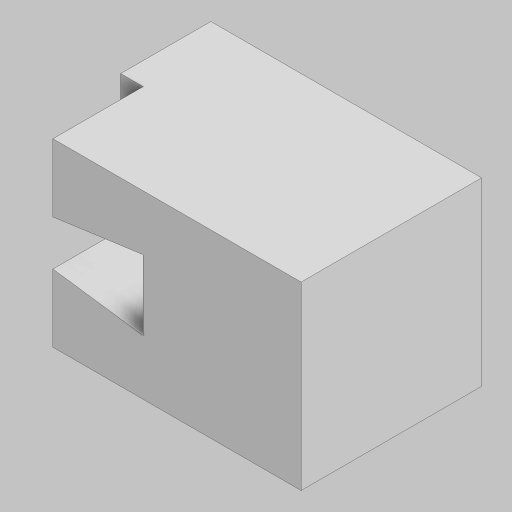
# Autodesk Inventor part: Hembra_parametrizada
Saved by Autodesk Inventor 2023 (Build 270158000, 158)
## iProperties
Created: 2026-02-22
Part Number: Hembra_parametrizada
Material: Genérico
Document SubType Name: Modeling
Designer: MARTIN MAESTRE
Density: 1 g/cm^3
Appearance: Valor por defecto
Author: MARTIN MAESTRE
Autodesk Inventor part; units mm, degrees
ref_plane "YZ Plane" through (0, 0, 0) normal (1, 0, 0) x (0, 1, 0)
ref_plane "XZ Plane" through (0, 0, 0) normal (0, 1, 0) x (-1, 0, 0)
ref_plane "XY Plane" through (0, 0, 0) normal (0, 0, 1) x (1, 0, 0)
sketch "Boceto1" plane through (0, 0, 0) normal (0, 0, 1) x (1, 0, 0)
  line L0 (0, 0) -> (60, 0)
  line L1 (60, 0) -> (60, 40)
  line L2 (60, 40) -> (0, 40)
  line L3 (0, 40) -> (0, 0)
  dimension "d0" = 60
  dimension "d1" = 40
  constraints: 8 end point, 2 parallel, 1 horizontal, 1 perpendicular
  measures "d0" distance of L2.end L1.end
  measures "d1" distance of L1.end L0.end
extrude "Extrusión1" add sketch "Boceto1" along normal blind 40
sketch "Boceto2" plane through (0, 0, 40) normal (0, 0, 1) x (1, 0, 0)
  line L0 (0, 40) -> (0, 0) projected
  line L1 (0, 0) -> (5, 0)
  line L2 (0, 0) -> (0, 40)
  line L3 (0, 40) -> (5, 40)
  line L4 (5, 0) -> (5, 15)
  line L5 (0, 0) -> (60, 0) projected
  line L6 (5, 0) -> (20, 0) construction
  line L7 (5, 40) -> (5, 25)
  line L8 (60, 40) -> (0, 40) projected
  line L9 (5, 40) -> (20, 40) construction
  line L10 (5, 40) -> (25, 40) construction
  line L11 (25, 40) -> (25, 27.75) construction
  line L12 (25, 40) -> (37.25, 40) construction
  line L13 (5, 0) -> (25, 0) construction
  line L14 (25, 0) -> (25, 12.25) construction
  line L15 (5, 25) -> (25, 27.75)
  line L16 (5, 15) -> (25, 12.25)
  line L17 (25, 27.75) -> (25, 12.25)
  dimension "d4" = 5
  dimension "d5" = 40
  dimension "d6" = 5
  dimension "d7" = 15
  dimension "d8" = 90
  dimension "d9" = 15
  dimension "d10" = 90
  dimension "d11" = 20
  dimension "d12" = 12.25
  dimension "d13" = 90
  dimension "d14" = 20
  dimension "d15" = 12.25
  dimension "d16" = 90
  constraints: 30 end point, 7 perpendicular, 4 horizontal, 2 point on line, 1 collinear, 1 vertical
  measures "d4" distance of L0.end L1.end
  measures "d5" distance of L0.end L0.start
  measures "d6" distance of L0.start L3.end
  measures "d7" distance of L1.end L4.end
  measures "d8" angle of L6 L4
  measures "d9" distance of L3.end L7.end
  measures "d10" angle of L7 L9
  measures "d11" distance of L3.end L10.end
  measures "d12" distance of L10.end L11.end
  measures "d13" angle of L11 L12
  measures "d14" distance of L1.end L13.end
  measures "d15" distance of L13.end L14.end
  measures "d16" angle of L14 L13
extrude "Extrusión2" cut sketch "Boceto2" against normal blind 20
equation "\"d4\" = Espesor_corte"
equation "\"d6\" = Espesor_corte"
equation "\"Espesor_corte\" = 5"
equation "\"Angulo_0\" = 0"
equation "\"Angulo_90\" = 90deg"
